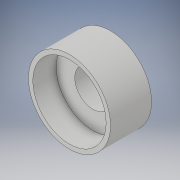
# Autodesk Inventor part: 30_raspi_lens_to_laser
Saved by Autodesk Inventor 2019 (Build 230136000, 136)
## iProperties
Created: 2020-09-01
Part Number: 30_raspi_lens_to_laser
Material: Generic
Document SubType Name: Modeling
Designer: marsikovabarbora
Density: 1 g/cm^3
Appearance: Default
Author: marsikovabarbora
Autodesk Inventor part; units mm, degrees
ref_plane "YZ Plane" through (0, 0, 0) normal (1, 0, 0) x (0, 1, 0)
ref_plane "XZ Plane" through (0, 0, 0) normal (0, 1, 0) x (-1, 0, 0)
ref_plane "XY Plane" through (0, 0, 0) normal (0, 0, 1) x (1, 0, 0)
sketch "Sketch1" plane through (0, 0, 0) normal (0, 0, 1) x (1, 0, 0)
  circle A0 centre (0, 0) radius 5.85 construction
  circle A1 centre (0, 0) radius 2.95 construction
  circle A2 centre (0, 0) radius 3.1
  circle A3 centre (0, 0) radius 7
  dimension "d0" = 11.7
  dimension "d1" = 5.9
  dimension "d2" = 6.2
  dimension "d3" = 14
  constraints: 4 centre point, 4 coincident
  measures "d0" diameter of A0
  measures "d1" diameter of A1
  measures "d2" diameter of A2
  measures "d3" diameter of A3
extrude "Extrusion1" add sketch "Sketch1" along normal blind 3
sketch "Sketch2" plane through (0, 0, 3) normal (0, 0, 1) x (1, 0, 0)
  circle A0 centre (0, 0) radius 5.85 construction
  circle A1 centre (0, 0) radius 2.95 construction
  circle A2 centre (0, 0) radius 7 projected
  circle A3 centre (0, 0) radius 6.25
  dimension "d6" = 11.7
  dimension "d7" = 5.9
  dimension "d10" = 12.5
  constraints: 3 centre point, 3 coincident
  measures "d6" diameter of A0
  measures "d7" diameter of A1
  measures "d10" diameter of A3
extrude "Extrusion2" add sketch "Sketch2" along normal blind 4
body "Solid1"
